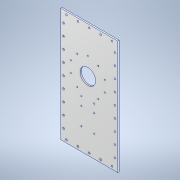
# Autodesk Inventor part: Podstawa
Saved by Autodesk Inventor 2022 (Build 260153000, 153)
## iProperties
Created: 2023-01-03
Part Number: Podstawa
Material: Aluminum 6061
Document SubType Name: Modeling
Designer: komputer
Density: 2.7 g/cm^3
Appearance: Aluminum - Flat
Author: komputer
Autodesk Inventor part; units mm, degrees
ref_plane "YZ Plane" through (0, 0, 0) normal (1, 0, 0) x (0, 1, 0)
ref_plane "XZ Plane" through (0, 0, 0) normal (0, 1, 0) x (-1, 0, 0)
ref_plane "XY Plane" through (0, 0, 0) normal (0, 0, 1) x (1, 0, 0)
sketch "Sketch1" plane through (0, 0, 0) normal (0, 0, 1) x (1, 0, 0)
  circle A0 centre (0, 0) radius 55 projected
  arc A1 (-1.4, -192.7776) -> (1.4, -192.7776) centre (0, -192.7776) ccw projected
  line L0 (-95, 160) -> (105, 160)
  line L1 (105, 160) -> (105, -240)
  line L2 (105, -240) -> (-95, -240)
  line L3 (-95, -240) -> (-95, 160)
  line L4 (-95, 200) -> (95, -200) construction
  line L5 (95, 200) -> (-95, -200) construction
  line L6 (0, 0) -> (0, -40) construction
  point P0 (0, 0)
  dimension "d58" = 200
  dimension "d59" = 400
  dimension "d60" = 40
  constraints: 14 end point, 2 midpoint, 2 parallel, 2 vertical, 1 horizontal, 1 perpendicular
  measures "d58" distance of L1.end L2.end
  measures "d59" distance of L0.end L1.end
  measures "d60" distance of L6.start L6.end
extrude "Extrusion1" add sketch "Sketch1" against normal blind 5
sketch "Sketch2" plane through (0, 0, 0) normal (0, 0, 1) x (1, 0, 0)
  circle A0 centre (-22.5, -100.6741) radius 2.25 projected
  circle A1 centre (22.5, -100.6741) radius 2.25 projected
  circle A2 centre (22.5, -71.1776) radius 2 projected
  circle A3 centre (-22.5, -71.1776) radius 2 projected
  circle A4 centre (-22.5, -162.7577) radius 2.25 projected
  circle A5 centre (22.5, -162.7577) radius 2.25 projected
  point P0 (0, 0)
  dimension "d53" = 71.1776
  dimension "d54" = 100.6741
  dimension "d55" = 162.7577
  measures "d53" vertical distance of point (0, 0) A2.centre
  measures "d54" vertical distance of point (0, 0) A1.centre
  measures "d55" vertical distance of point (0, 0) A5.centre
hole "Hole1" at (22.5, -71.1776, 0) at (-22.5, -71.1776, 0) at (-22.5, -100.6741, 0) at (22.5, -100.6741, 0) at (-22.5, -162.7577, 0) at (22.5, -162.7577, 0) direction (0, 0, -1) diameter 4 end through all
sketch "Sketch3" plane through (0, 0, 0) normal (0, 0, 1) x (1, 0, 0)
  line L0 (1.9053, 65.8) -> (3.8105, 62.5) projected
  line L1 (-1.9053, 65.8) -> (1.9053, 65.8) projected
  line L2 (-3.8105, 62.5) -> (-1.9053, 65.8) projected
  line L3 (-1.9053, 59.2) -> (-3.8105, 62.5) projected
  line L4 (1.9053, 59.2) -> (-1.9053, 59.2) projected
  line L5 (3.8105, 62.5) -> (1.9053, 59.2) projected
  line L6 (-33.2555, 49.0137) -> (-36.3383, 46.7739) projected
  line L7 (-33.6538, 52.8033) -> (-33.2555, 49.0137) projected
  line L8 (-37.1349, 54.3532) -> (-33.6538, 52.8033) projected
  line L9 (-40.2177, 52.1134) -> (-37.1349, 54.3532) projected
  line L10 (-39.8193, 48.3238) -> (-40.2177, 52.1134) projected
  line L11 (-36.3383, 46.7739) -> (-39.8193, 48.3238) projected
  line L12 (-55.7138, 20.1058) -> (-56.8913, 16.4818) projected
  line L13 (-58.2635, 22.9376) -> (-55.7138, 20.1058) projected
  line L14 (-61.9908, 22.1453) -> (-58.2635, 22.9376) projected
  line L15 (-63.1683, 18.5213) -> (-61.9908, 22.1453) projected
  line L16 (-60.6185, 15.6896) -> (-63.1683, 18.5213) projected
  line L17 (-56.8913, 16.4818) -> (-60.6185, 15.6896) projected
  line L18 (-56.8913, -16.4818) -> (-55.7138, -20.1058) projected
  line L19 (-60.6185, -15.6896) -> (-56.8913, -16.4818) projected
  line L20 (-63.1683, -18.5213) -> (-60.6185, -15.6896) projected
  line L21 (-61.9908, -22.1453) -> (-63.1683, -18.5213) projected
  line L22 (-58.2635, -22.9376) -> (-61.9908, -22.1453) projected
  line L23 (-55.7138, -20.1058) -> (-58.2635, -22.9376) projected
  line L24 (-36.3383, -46.7739) -> (-33.2555, -49.0137) projected
  line L25 (-39.8193, -48.3238) -> (-36.3383, -46.7739) projected
  line L26 (-40.2177, -52.1134) -> (-39.8193, -48.3238) projected
  line L27 (-37.1349, -54.3532) -> (-40.2177, -52.1134) projected
  line L28 (-33.6538, -52.8033) -> (-37.1349, -54.3532) projected
  line L29 (-33.2555, -49.0137) -> (-33.6538, -52.8033) projected
  line L30 (33.2555, -49.0137) -> (36.3383, -46.7739) projected
  line L31 (33.6538, -52.8033) -> (33.2555, -49.0137) projected
  line L32 (37.1349, -54.3532) -> (33.6538, -52.8033) projected
  line L33 (40.2177, -52.1134) -> (37.1349, -54.3532) projected
  line L34 (39.8193, -48.3238) -> (40.2177, -52.1134) projected
  line L35 (36.3383, -46.7739) -> (39.8193, -48.3238) projected
  line L36 (55.7138, -20.1058) -> (56.8913, -16.4818) projected
  line L37 (58.2635, -22.9376) -> (55.7138, -20.1058) projected
  line L38 (61.9908, -22.1453) -> (58.2635, -22.9376) projected
  line L39 (63.1683, -18.5213) -> (61.9908, -22.1453) projected
  line L40 (60.6185, -15.6896) -> (63.1683, -18.5213) projected
  line L41 (56.8913, -16.4818) -> (60.6185, -15.6896) projected
  line L42 (56.8913, 16.4818) -> (55.7138, 20.1058) projected
  line L43 (60.6185, 15.6896) -> (56.8913, 16.4818) projected
  line L44 (63.1683, 18.5213) -> (60.6185, 15.6896) projected
  line L45 (61.9908, 22.1453) -> (63.1683, 18.5213) projected
  line L46 (58.2635, 22.9376) -> (61.9908, 22.1453) projected
  line L47 (55.7138, 20.1058) -> (58.2635, 22.9376) projected
  line L48 (36.3383, 46.7739) -> (33.2555, 49.0137) projected
  line L49 (39.8193, 48.3238) -> (36.3383, 46.7739) projected
  line L50 (40.2177, 52.1134) -> (39.8193, 48.3238) projected
  line L51 (37.1349, 54.3532) -> (40.2177, 52.1134) projected
  line L52 (33.6538, 52.8033) -> (37.1349, 54.3532) projected
  line L53 (33.2555, 49.0137) -> (33.6538, 52.8033) projected
  circle A0 centre (0, 0) radius 42 projected
  line L54 (1.9053, 65.8) -> (-1.9053, 59.2)
  line L55 (-3.8105, 62.5) -> (3.8105, 62.5)
  arc A1 (41.8018, -53.634) -> (-41.8018, -53.634) centre (0, 0) ccw projected
  arc A2 (31.3377, -53) -> (41.8018, -53.634) centre (36.7366, -50.5636) ccw projected
  line L56 (-31.3377, -53) -> (31.3377, -53) projected
  arc A3 (-41.8018, -53.634) -> (-31.3377, -53) centre (-36.7366, -50.5636) ccw projected
  point P0 (0, 0)
  point P1 (0, 62.5)
  point P2 (-36.7366, 50.5636)
  point P3 (0, 0)
  point P4 (-59.441, 19.3136)
  point P5 (0, 0)
  point P6 (-59.441, -19.3136)
  point P7 (0, 0)
  point P8 (-36.7366, -50.5636)
  point P9 (0, 0)
  point P10 (0, -62.5)
  point P11 (0, 0)
  point P12 (36.7366, -50.5636)
  point P13 (0, 0)
  point P14 (59.441, -19.3136)
  point P15 (0, 0)
  point P16 (59.441, 19.3136)
  point P17 (0, 0)
  point P18 (36.7366, 50.5636)
  point P19 (0, 0)
  constraints: 4 end point, 1 midpoint, 1 point on line
hole "Hole2" at (0, 62.5, 0) at (-36.7366, 50.5636, 0) at (-59.441, 19.3136, 0) at (-59.441, -19.3136, 0) at (-36.7366, -50.5636, 0) at (0, -62.5, 0) at (36.7366, -50.5636, 0) at (59.441, -19.3136, 0) at (59.441, 19.3136, 0) at (36.7366, 50.5636, 0) direction (0, 0, -1) diameter 4 end through all
sketch "Sketch4" plane through (0, 0, 0) normal (0, 0, 1) x (1, 0, 0)
  circle A0 centre (-2.7145, -65.4202) radius 7.4729
  point P0 (0, 0)
  constraints: 1 centre point
extrude "Extrusion2" add sketch "Sketch4" against normal blind 5
sketch "Sketch6" plane through (0, 0, 0) normal (0, 0, 1) x (1, 0, 0)
  circle A0 centre (0, 0) radius 27.5
  circle A1 centre (59.441, 19.3136) radius 2 projected
  circle A2 centre (36.7366, -50.5636) radius 2 projected
  circle A3 centre (-36.7366, -50.5636) radius 2 projected
  circle A4 centre (-59.441, 19.3136) radius 2 projected
  circle A5 centre (0, 62.5) radius 2 projected
  circle A6 centre (-36.7366, 50.5636) radius 2 projected
  circle A7 centre (-59.441, -19.3136) radius 2 projected
  circle A8 centre (59.441, -19.3136) radius 2 projected
  circle A9 centre (36.7366, 50.5636) radius 2 projected
  circle A10 centre (-22.5, -162.7577) radius 2 projected
  circle A11 centre (-22.5, -100.6741) radius 2 projected
  circle A12 centre (22.5, -71.1776) radius 2 projected
  circle A13 centre (-22.5, -71.1776) radius 2 projected
  circle A14 centre (22.5, -100.6741) radius 2 projected
  circle A15 centre (22.5, -162.7577) radius 2 projected
  circle A16 centre (0, 0) radius 55 projected
  dimension "d38" = 55
  constraints: 1 centre point, 1 coincident
  measures "d38" diameter of A0
extrude "Extrusion3" add sketch "Sketch6" against normal up to surface (5 mm away) contours A16
sketch "Sketch9" plane through (0, 0, 0) normal (0, 0, 1) x (1, 0, 0)
  circle A0 centre (0, 0) radius 27.5 projected
  circle A1 centre (59.441, 19.3136) radius 2 projected
  circle A2 centre (36.7366, -50.5636) radius 2 projected
  circle A3 centre (-36.7366, -50.5636) radius 2 projected
  circle A4 centre (-59.441, 19.3136) radius 2 projected
  circle A5 centre (0, 62.5) radius 2 projected
  circle A6 centre (-36.7366, 50.5636) radius 2 projected
  circle A7 centre (-59.441, -19.3136) radius 2 projected
  circle A8 centre (59.441, -19.3136) radius 2 projected
  circle A9 centre (36.7366, 50.5636) radius 2 projected
  circle A10 centre (-22.5, -162.7577) radius 2 projected
  circle A11 centre (-22.5, -100.6741) radius 2 projected
  circle A12 centre (22.5, -71.1776) radius 2 projected
  circle A13 centre (-22.5, -71.1776) radius 2 projected
  circle A14 centre (22.5, -100.6741) radius 2 projected
  circle A15 centre (22.5, -162.7577) radius 2 projected
  line L0 (-95, -240) -> (105, -240) projected
  line L1 (105, -240) -> (105, 160) projected
  line L2 (105, 160) -> (-95, 160) projected
  line L3 (-95, 160) -> (-95, -240) projected
  line L4 (-85, -230) -> (95, -230) construction
  line L5 (95, -230) -> (95, 150) construction
  line L6 (95, 150) -> (-85, 150) construction
  line L7 (-85, 150) -> (-85, -230) construction
  line L8 (-95, -240) -> (-95, 160) construction
  line L9 (-95, -230) -> (-75, -230) construction
  point P0 (-35, -230)
  point P1 (5, -230)
  point P2 (45, -230)
  point P3 (85, -230)
  point P4 (-75, 150)
  point P5 (-35, 150)
  point P6 (5, 150)
  point P7 (45, 150)
  point P8 (85, 150)
  dimension "d61" = 10
  dimension "d62" = 20
  dimension "d65" = 40
  dimension "d68" = 380
  constraints: 10 end point, 2 point on line, 1 coincident, 1 horizontal, 1 vertical, 12 other
  measures "d61" distance between parallel lines of L3 L7
  measures "d62" distance of L9.start L9.end
  measures "d65" distance of point (-75, -230) point (-35, -230)
  measures "d68" distance of point (-75, -230) point (-75, 150)
hole "Hole4" at (-75, -230, 0) at (-35, -230, 0) at (5, -230, 0) at (45, -230, 0) at (85, -230, 0) at (-75, 150, 0) at (-35, 150, 0) at (5, 150, 0) at (45, 150, 0) at (85, 150, 0) direction (0, 0, -1) diameter 6 end through all
sketch "Sketch10" plane through (0, 0, 0) normal (0, 0, 1) x (1, 0, 0)
  circle A0 centre (45, 150) radius 3 projected
  circle A1 centre (-35, 150) radius 3 projected
  circle A2 centre (85, -230) radius 3 projected
  circle A3 centre (5, -230) radius 3 projected
  circle A4 centre (-75, -230) radius 3 projected
  circle A5 centre (-35, -230) radius 3 projected
  circle A6 centre (45, -230) radius 3 projected
  circle A7 centre (-75, 150) radius 3 projected
  circle A8 centre (5, 150) radius 3 projected
  circle A9 centre (85, 150) radius 3 projected
  circle A10 centre (0, 0) radius 27.5 projected
  circle A11 centre (59.441, 19.3136) radius 2 projected
  circle A12 centre (36.7366, -50.5636) radius 2 projected
  circle A13 centre (-36.7366, -50.5636) radius 2 projected
  circle A14 centre (-59.441, 19.3136) radius 2 projected
  circle A15 centre (0, 62.5) radius 2 projected
  circle A16 centre (-36.7366, 50.5636) radius 2 projected
  circle A17 centre (-59.441, -19.3136) radius 2 projected
  circle A18 centre (59.441, -19.3136) radius 2 projected
  circle A19 centre (36.7366, 50.5636) radius 2 projected
  circle A20 centre (-22.5, -162.7577) radius 2 projected
  circle A21 centre (-22.5, -100.6741) radius 2 projected
  circle A22 centre (22.5, -71.1776) radius 2 projected
  circle A23 centre (-22.5, -71.1776) radius 2 projected
  circle A24 centre (22.5, -100.6741) radius 2 projected
  circle A25 centre (22.5, -162.7577) radius 2 projected
  line L0 (-95, -240) -> (105, -240) projected
  line L1 (105, -240) -> (105, 160) projected
  line L2 (105, 160) -> (-95, 160) projected
  line L3 (-95, 160) -> (-95, -240) projected
  line L4 (-85, -230) -> (95, -230)
  line L5 (95, -230) -> (95, 150)
  line L6 (95, 150) -> (-85, 150)
  line L7 (-85, 150) -> (-85, -230)
  line L8 (-85, -230) -> (-85, -200)
  point P0 (-85, -160)
  point P1 (-85, -120)
  point P2 (-85, -80)
  point P3 (-85, -40)
  point P4 (-85, 0)
  point P5 (-85, 40)
  point P6 (-85, 80)
  point P7 (-85, 120)
  point P8 (95, -200)
  point P9 (95, -160)
  point P10 (95, -120)
  point P11 (95, -80)
  point P12 (95, -40)
  point P13 (95, 0)
  point P14 (95, 40)
  point P15 (95, 80)
  point P16 (95, 120)
  dimension "d78" = 10
  dimension "d79" = 30
  dimension "d82" = 40
  dimension "d85" = 180
  constraints: 10 end point, 1 coincident, 1 horizontal, 1 point on line, 1 vertical, 20 other
  measures "d78" distance between parallel lines of L3 L7
  measures "d79" distance of L4.start L8.end
  measures "d82" distance of point (-85, -200) point (-85, -160)
  measures "d85" distance of point (-85, -200) point (95, -200)
hole "Hole5" at (-85, -200, 0) at (-85, -160, 0) at (-85, -120, 0) at (-85, -80, 0) at (-85, -40, 0) at (-85, 0, 0) at (-85, 40, 0) at (-85, 80, 0) at (-85, 120, 0) at (95, -200, 0) at (95, -160, 0) at (95, -120, 0) at (95, -80, 0) at (95, -40, 0) at (95, 0, 0) at (95, 40, 0) at (95, 80, 0) at (95, 120, 0) direction (0, 0, -1) diameter 6 end through all
body "Solid1"
